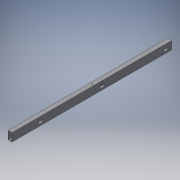
# Autodesk Inventor part: 41.75in Arm Beam Alternate (Right)
Saved by Autodesk Inventor 2018.3 (Build 223284000, 284)
## iProperties
Created: 2019-01-17
Part Number: 41.75in Arm Beam Alternate (Right)
Material: Generic
Document SubType Name: Modeling
Designer: Gabriel
Density: 1 g/cm^3
Appearance: Default
Author: Gabriel
Autodesk Inventor part; units mm, degrees
ref_plane "YZ Plane" through (0, 0, 0) normal (1, 0, 0) x (0, 1, 0)
ref_plane "XZ Plane" through (0, 0, 0) normal (0, 1, 0) x (-1, 0, 0)
ref_plane "XY Plane" through (0, 0, 0) normal (0, 0, 1) x (1, 0, 0)
sketch "Sketch1" plane through (0, 0, 0) normal (0, 0, 1) x (1, 0, 0)
  line L0 (-35.3228, 16.049) -> (-9.9228, 16.049)
  line L1 (-9.9228, 16.049) -> (-9.9228, -34.751)
  line L2 (-9.9228, -34.751) -> (-35.3228, -34.751)
  line L3 (-35.3228, -34.751) -> (-35.3228, 16.049)
  line L4 (-13.0978, 12.874) -> (-32.1478, 12.874)
  line L5 (-32.1478, 12.874) -> (-32.1478, -31.576)
  line L6 (-32.1478, -31.576) -> (-13.0978, -31.576)
  line L7 (-13.0978, -31.576) -> (-13.0978, 12.874)
  point P0 (0, 0)
  dimension "d0" = 25.4
  dimension "d1" = 50.8
  dimension "d2" = 3.175
  constraints: 16 end point, 4 parallel, 2 perpendicular, 1 horizontal, 3 other
  measures "d0" distance of L1.end L2.end
  measures "d1" distance of L0.end L1.end
  measures "d2" distance between parallel lines of L0 L4
extrude "Extrusion1" add sketch "Sketch1" along normal blind 977.9
sketch "Sketch2" plane through (-35.3228, -34.751, 0) normal (-1, 0, 0) x (0, 0, 1)
  line L0 (0, 0) -> (0, 50.8) construction
  line L1 (0, 25.4) -> (25.4, 25.4) construction
  circle A0 centre (25.4, 25.4) radius 12.7
  point P0 (0, 34.751)
  dimension "d5" = 25.4
  dimension "d9" = 25.4
  constraints: 2 end point, 1 centre point, 1 coincident, 1 horizontal, 1 midpoint
  measures "d5" distance of L1.start L1.end
  measures "d9" diameter of A0
extrude "Extrusion2" cut sketch "Sketch2" against normal blind 12.7
sketch "Sketch3" plane through (-35.3228, -34.751, 0) normal (-1, 0, 0) x (0, 0, 1)
  line L0 (977.9, 50.8) -> (977.9, 0) construction
  line L1 (977.9, 25.4) -> (800.1, 25.4) construction
  circle A0 centre (800.1, 25.4) radius 14.2875
  point P0 (0, 34.751)
  dimension "d10" = 177.8
  dimension "d11" = 28.575
  constraints: 2 end point, 1 centre point, 1 coincident, 1 horizontal, 1 midpoint
  measures "d10" distance of L1.start L1.end
  measures "d11" diameter of A0
extrude "Extrusion3" cut sketch "Sketch3" against normal blind 25.4
sketch "Sketch4" plane through (-35.3228, -34.751, 0) normal (-1, 0, 0) x (0, 0, 1)
  line L0 (977.9, 50.8) -> (977.9, 0) construction
  line L1 (977.9, 25.4) -> (419.1, 25.4) construction
  circle A0 centre (419.1, 25.4) radius 14.2875
  point P0 (0, 34.751)
  dimension "d14" = 558.8
  dimension "d15" = 28.575
  constraints: 2 end point, 1 centre point, 1 coincident, 1 horizontal, 1 midpoint
  measures "d14" distance of L1.start L1.end
  measures "d15" diameter of A0
extrude "Extrusion4" cut sketch "Sketch4" against normal blind 25.4
sketch "Sketch5" plane through (-35.3228, -34.751, 0) normal (-1, 0, 0) x (0, 0, 1)
  circle A0 centre (419.1, 25.4) radius 14.2875 construction
  line L0 (419.1, 25.4) -> (401.1395, 7.4395) construction
  line L1 (419.1, 25.4) -> (444.5, 25.4) construction
  line L2 (419.1, 25.4) -> (437.0605, 43.3605) construction
  circle A1 centre (401.1395, 7.4395) radius 2.032
  circle A2 centre (437.0605, 43.3605) radius 2.032
  point P0 (0, 34.751)
  dimension "d18" = 25.4
  dimension "d19" = 135
  dimension "d20" = 25.4
  dimension "d21" = 4.064
  dimension "d22" = 4.064
  constraints: 6 end point, 2 centre point, 2 coincident, 1 equal length, 1 horizontal
  measures "d18" distance of L0.start L0.end
  measures "d19" angle of L0 L1
  measures "d20" distance of L0.start L2.end
  measures "d21" diameter of A1
  measures "d22" diameter of A2
extrude "Extrusion5" cut sketch "Sketch5" against normal blind 25.4
sketch "Sketch7" plane through (-9.9228, -34.751, 0) normal (1, 0, 0) x (0, 0, -1)
  line L0 (0, 0) -> (0, 50.8) construction
  line L1 (0, 25.4) -> (-25.4, 25.4) construction
  circle A0 centre (-25.4, 25.4) radius 14.2875
  point P0 (0, 34.751)
  dimension "d34" = 25.4
  dimension "d35" = 28.575
  constraints: 2 end point, 1 centre point, 1 coincident, 1 horizontal, 1 midpoint
  measures "d34" distance of L1.start L1.end
  measures "d35" diameter of A0
extrude "Extrusion7" cut sketch "Sketch7" against normal blind 12.7
sketch "Sketch8" plane through (-9.9228, -34.751, 0) normal (1, 0, 0) x (0, 0, -1)
  circle A0 centre (-25.4, 25.4) radius 14.2875 construction
  line L0 (-25.4, 25.4) -> (-25.4, 49.2125) construction
  line L1 (-25.4, 49.2125) -> (-4.7778, 37.3063) construction
  line L2 (-4.7778, 37.3063) -> (-4.7778, 13.4938) construction
  line L3 (-4.7778, 13.4938) -> (-25.4, 1.5875) construction
  line L4 (-25.4, 1.5875) -> (-46.0222, 13.4937) construction
  line L5 (-46.0222, 13.4937) -> (-46.0222, 37.3062) construction
  line L6 (-46.0222, 37.3062) -> (-25.4, 49.2125) construction
  circle A1 centre (-4.7778, 37.3063) radius 2.5797
  circle A2 centre (-4.7778, 13.4938) radius 2.5797
  circle A3 centre (-46.0222, 13.4937) radius 2.5797
  circle A4 centre (-46.0222, 37.3062) radius 2.5797
  point P0 (0, 34.751)
  dimension "d45" = 23.8125
  dimension "d46" = 5.1594
  dimension "d47" = 5.1594
  dimension "d48" = 5.1594
  dimension "d49" = 5.1594
  constraints: 14 end point, 5 coincident, 4 centre point, 1 vertical, 13 other
  measures "d45" distance of L0.start L0.end
  measures "d46" diameter of A1
  measures "d47" diameter of A2
  measures "d48" diameter of A3
  measures "d49" diameter of A4
extrude "Extrusion9" cut sketch "Sketch8" against normal blind 25.4
sketch "Sketch9" plane through (0, 0, 0) normal (0, 0, -1) x (-1, 0, 0)
  line L0 (9.9228, 16.049) -> (35.3228, 16.049) projected
  line L1 (9.9228, 16.049) -> (13.0978, 16.049)
  line L2 (13.0978, 16.049) -> (13.0978, -34.751)
  line L3 (13.0978, -34.751) -> (9.9228, -34.751)
  line L4 (9.9228, -34.751) -> (9.9228, 16.049)
  line L5 (9.9228, -34.751) -> (35.3228, -34.751)
  line L6 (35.3228, -34.751) -> (35.3228, -31.576)
  line L7 (35.3228, -31.576) -> (9.9228, -31.576)
  line L8 (9.9228, -31.576) -> (9.9228, -34.751)
  line L9 (9.9228, -34.751) -> (35.3228, -34.751) projected
  line L10 (35.3228, -34.751) -> (32.1478, -34.751)
  line L11 (32.1478, -34.751) -> (32.1478, 16.049)
  line L12 (32.1478, 16.049) -> (35.3228, 16.049)
  line L13 (35.3228, 16.049) -> (35.3228, -34.751)
  line L14 (35.3228, 16.049) -> (9.9228, 16.049)
  line L15 (9.9228, 16.049) -> (9.9228, 12.874)
  line L16 (9.9228, 12.874) -> (35.3228, 12.874)
  line L17 (35.3228, 12.874) -> (35.3228, 16.049)
  point P0 (0, 0)
  dimension "d52" = 3.175
  dimension "d53" = 50.8
  dimension "d54" = 25.4
  dimension "d55" = 3.175
  dimension "d56" = 3.175
  dimension "d57" = 50.8
  dimension "d58" = 25.4
  dimension "d59" = 3.175
  constraints: 32 end point, 8 parallel, 4 horizontal, 4 perpendicular
  measures "d52" distance of L2.end L3.end
  measures "d53" distance of L1.end L2.end
  measures "d54" distance of L7.end L6.end
  measures "d55" distance of L6.end L5.end
  measures "d56" distance of L11.end L12.end
  measures "d57" distance of L10.end L11.end
  measures "d58" distance of L16.end L15.end
  measures "d59" distance of L15.end L14.end
extrude "Extrusion10" add sketch "Sketch9" along normal blind 12.7 contours L0 L2 L16 L4 | L0 L11 L16 L2 | L16 L2 L7 L4 | L0 L13 L16 L11 | L7 L2 L3 L4 | L16 L13 L7 L11 | L7 L11 L5 L2 | L7 L6 L5 L11
sketch "Sketch10" plane through (-35.3228, 16.049, 977.9) normal (0, 1, 0) x (1, 0, 0)
  line L0 (3.175, 0) -> (22.225, 0) construction
  line L1 (12.7, 0) -> (12.7, 508) construction
  line L2 (12.7, 0) -> (520.7, 0) construction
  circle A0 centre (12.7, 508) radius 2.5797
  point P0 (35.3228, 977.9)
  dimension "d62" = 508
  dimension "d63" = 90
  dimension "d64" = 5.1594
  constraints: 4 end point, 1 centre point, 1 coincident, 1 horizontal, 1 midpoint, 1 perpendicular, 1 vertical
  measures "d62" distance of L1.start L1.end
  measures "d63" angle of L2 L1
  measures "d64" diameter of A0
extrude "Extrusion11" cut sketch "Sketch10" against normal blind 101.6
body "Solid1"
